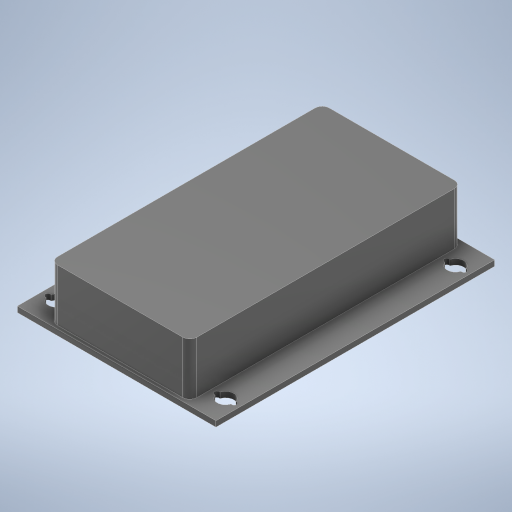
# Autodesk Inventor part: SUSTAINA-POWER-MONITOR-BOARD1
Saved by Autodesk Inventor 2024.2 (Build 282272000, 272)
## iProperties
Created: 2024-01-24
Part Number: SUSTAINA-POWER-MONITOR-BOARD1
Material: Acetal Resin, Black
Document SubType Name: Modeling
Designer: Masato Kubotera
Appearance: Smooth - Black
Surface Area: 123.153 cm^2
Volume: 52.2328 cm^3
Author: Masato Kubotera
Autodesk Inventor part; units mm, degrees
ref_plane "YZ Plane" through (0, 0, 0) normal (1, 0, 0) x (0, 1, 0)
ref_plane "XZ Plane" through (0, 0, 0) normal (0, 1, 0) x (-1, 0, 0)
ref_plane "XY Plane" through (0, 0, 0) normal (0, 0, 1) x (1, 0, 0)
sketch "Sketch1" plane through (0, 0, 0) normal (0, 0, 1) x (1, 0, 0)
  line L0 (40, 28.5) -> (-40, 28.5)
  line L1 (-40, 28.5) -> (-40, -28.5)
  line L2 (-40, -28.5) -> (40, -28.5)
  line L3 (40, -28.5) -> (40, 28.5)
  line L4 (40, 28.5) -> (-40, -28.5) construction
  line L5 (-40, 28.5) -> (40, -28.5) construction
  line L6 (-33, 24.25) -> (33, 24.25) construction
  line L7 (33, 24.25) -> (33, -24.25) construction
  line L8 (33, -24.25) -> (-33, -24.25) construction
  line L9 (-33, -24.25) -> (-33, 24.25) construction
  line L10 (-33, 24.25) -> (33, -24.25) construction
  line L11 (33, 24.25) -> (-33, -24.25) construction
  line L12 (40, 0) -> (-40, 0) construction
  line L13 (0, 28.5) -> (0, -28.5) construction
  circle A0 centre (33, 24.25) radius 2.4
  circle A1 centre (-33, 24.25) radius 2.4
  circle A2 centre (33, -24.25) radius 2.4
  circle A3 centre (-33, -24.25) radius 2.4
  line L14 (33, 27.5) -> (33, 21) construction
  arc A4 (32.2801, 21.9605) -> (33.7199, 21.9605) centre (33, 21.75) ccw
  arc A5 (-33.7199, 21.9605) -> (-32.2801, 21.9605) centre (-33, 21.75) ccw
  arc A6 (33.7199, -21.9605) -> (32.2801, -21.9605) centre (33, -21.75) ccw
  arc A7 (-32.2801, -21.9605) -> (-33.7199, -21.9605) centre (-33, -21.75) ccw
  line L15 (39, 20) -> (-39, 20)
  line L16 (-39, 20) -> (-39, -20)
  line L17 (-39, -20) -> (39, -20)
  line L18 (39, -20) -> (39, 20)
  line L19 (39, 20) -> (-39, -20) construction
  line L20 (-39, 20) -> (39, -20) construction
  arc A8 (33.7199, 26.5395) -> (32.2801, 26.5395) centre (33, 26.75) ccw
  arc A9 (-32.2801, 26.5395) -> (-33.7199, 26.5395) centre (-33, 26.75) ccw
  arc A10 (32.2801, -26.5395) -> (33.7199, -26.5395) centre (33, -26.75) ccw
  arc A11 (-33.7199, -26.5395) -> (-32.2801, -26.5395) centre (-33, -26.75) ccw
  point P0 (0, 0)
  point P1 (33, 21)
  point P2 (33, -21)
  point P3 (-32.2801, 21.9605)
  point P4 (-33.7199, 21.9605)
  point P5 (-33.7199, -21.9605)
  point P6 (-32.2801, -21.9605)
  point P7 (32.2801, -21.9605)
  point P8 (33.7199, -21.9605)
  point P9 (33, 27.5)
  point P10 (32.2801, 26.5395)
  point P11 (33.7199, 26.5395)
  point P12 (-33.7199, 26.5395)
  point P13 (-32.2801, 26.5395)
  point P14 (-32.2801, -26.5395)
  point P15 (-33.7199, -26.5395)
  point P16 (33.7199, -26.5395)
  point P17 (32.2801, -26.5395)
  dimension "d0" = 80
  dimension "d1" = 57
  dimension "d19" = 4.8
  dimension "d30" = 6.5
  dimension "d33" = 48.5
  dimension "d34" = 66
  dimension "d36" = 1.5
  dimension "d37" = 8.5
  dimension "d38" = 1
  dimension "d41" = 14
  dimension "d42" = 6.5
  dimension "d43" = 1
  constraints: 42 end point, 25 symmetric about line, 20 point on circle, 12 centre point, 11 midpoint, 6 coincident, 6 parallel, 3 horizontal, 3 perpendicular, 1 point on line, 1 vertical, 11 other
  measures "d0" distance of L2.end L1.end
  measures "d1" distance of L1.end L0.end
  measures "d19" diameter of A0
  measures "d30" distance of L14.start L14.end
  measures "d33" distance of L8.end L6.start
  measures "d34" distance of L7.end L8.end
  measures "d36" diameter of A4
  measures "d37" diameter of L0 L6
  measures "d38" distance between parallel lines of L3 L18
  measures "d41" diameter of L3 L7
  measures "d42" distance of point (33, 27.5) point (33, 21)
  measures "d43" distance from line of L0 L14.start
extrude "Extrusion1" add sketch "Sketch1" along normal blind 1.6 contours L3 L2 L1 L0 | L18 L17 L16 L15
extrude "Extrusion2" add sketch "Sketch1" along normal blind 16.6 contours L18 L17 L16 L15
fillet "Fillet1" radius 2 4 edges at (39, -20, 9.1) (39, 20, 9.1) (-39, -20, 9.1) (-39, 20, 9.1)
body "Solid1"
